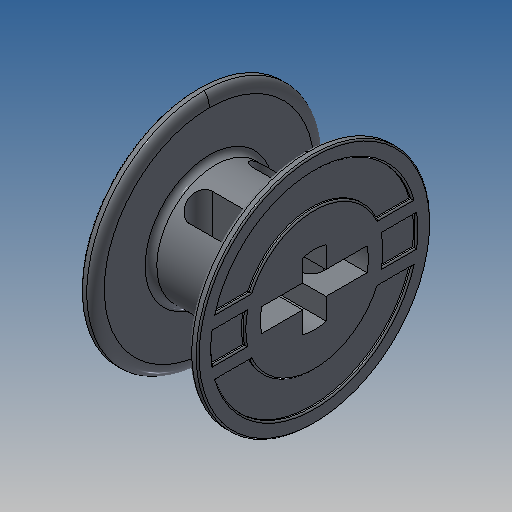
# Autodesk Inventor part: 61510-LtBluishGray
Saved by Autodesk Inventor 2025 (Build 290162010, 162A)
## iProperties
Created: 2014-10-31
Part Number: 61510-LtBluishGray
Material: ABS Plastic
Document SubType Name: Modeling
Designer: D. Kohfeld
Density: 1.06 g/cm^3
Appearance: LtBluishGray
Mass: 0.428094 g
Surface Area: 11.3807 cm^2
Volume: 0.403862 cm^3
Author: D. Kohfeld
Autodesk Inventor part; units mm, degrees
ref_plane "YZ Plane" through (0, 0, 0) normal (1, 0, 0) x (0, 1, 0)
ref_plane "XZ Plane" through (0, 0, 0) normal (0, 1, 0) x (-1, 0, 0)
ref_plane "XY Plane" through (0, 0, 0) normal (0, 0, 1) x (1, 0, 0)
sketch "Sketch2" plane through (0, 0, 0) normal (0, 0, 1) x (1, 0, 0)
  line L0 (-4, 8) -> (-4, 7)
  line L1 (-4, 7) -> (-3.8, 7)
  line L2 (-3.8, 7) -> (-3.8, 4.8)
  line L3 (-3.8, 4.8) -> (-4, 4.8)
  line L4 (-4, 4.8) -> (-4, 0)
  line L5 (-4, 0) -> (4, 0)
  line L6 (4, 0) -> (4, 4.8)
  line L7 (4, 4.8) -> (3.8, 4.8)
  line L8 (3.8, 4.8) -> (3.8, 7)
  line L9 (3.8, 7) -> (4, 7)
  line L10 (4, 7) -> (4, 8)
  line L11 (4, 8) -> (3.6, 8)
  line L12 (3.2, 7.2) -> (3.2, 4.4)
  arc A0 (2.8, 4) -> (3.2, 4.4) centre (2.8, 4.4) ccw
  line L13 (2.8, 4) -> (-2.8, 4)
  arc A1 (-3.2, 4.4) -> (-2.8, 4) centre (-2.8, 4.4) ccw
  line L14 (-3.2, 4.4) -> (-3.2, 7.2)
  line L15 (-3.6, 8) -> (-4, 8)
  ellipse E0 centre (-3.6, 7.2) end of major axis (-3.6, 8) minor radius 0.4 (-3.2, 7.2) -> (-3.6, 8) ccw
  ellipse E1 centre (3.6, 7.2) end of major axis (3.6, 8) minor radius 0.4 (3.6, 8) -> (3.2, 7.2) ccw
  point P0 (0, 0)
  point P1 (0, 0)
  dimension "d0" = 16
  dimension "d1" = 8
  dimension "d2" = 0.2
  dimension "d3" = 9.6
  dimension "d4" = 14
  dimension "d5" = 0.8
  dimension "d6" = 8
  dimension "d7" = 0.4
  dimension "d8" = 0.8
  dimension "d9" = 0.8
  dimension "d10" = 0.4
  constraints: 32 end point, 12 parallel, 4 equal length, 4 horizontal alignment, 4 point on circle, 4 tangent, 4 vertical alignment, 3 vertical, 2 centre point, 2 collinear, 1 coincident, 1 equal radius, 1 midpoint, 1 perpendicular, 8 other
  measures "d0" diameter of L15 L5
  measures "d1" distance between parallel lines of L10 L0
  measures "d2" distance between parallel lines of L0 L2
  measures "d3" diameter of L3.end L5
  measures "d4" diameter of L0.end L5
  measures "d5" distance between parallel lines of L14 L0
  measures "d6" diameter of L13 L5
  measures "d7" distance from line of L15.start L0
  measures "d8" distance from line of L14.end L15
  measures "d9" distance between parallel lines of L12 L10
  measures "d10" radius of A1
revolve "Revolution1" add sketch "Sketch2" angle 360 about axis through (-4, 0, 0) along (1, 0, 0)
sketch "Sketch3" plane through (4, 0, 0) normal (1, 0, 0) x (0, 0, -1)
  circle A0 centre (0, 0) radius 4.8 projected
  circle A1 centre (0, 0) radius 2.4 construction
  line L0 (-0.8, 2.2627) -> (-0.8, 0.8)
  line L1 (-0.8, 0.8) -> (-3.6125, 0.8)
  line L2 (0.8, 2.2627) -> (0.8, 0.8)
  line L3 (0.8, 0.8) -> (3.6125, 0.8)
  line L4 (-0.8, -2.2627) -> (-0.8, -0.8)
  line L5 (-0.8, -0.8) -> (-3.6125, -0.8)
  line L6 (0.8, -2.2627) -> (0.8, -0.8)
  line L7 (0.8, -0.8) -> (3.6125, -0.8)
  arc A2 (-3.6125, 0.8) -> (-3.6125, -0.8) centre (0, 0) ccw
  arc A3 (3.6125, -0.8) -> (3.6125, 0.8) centre (0, 0) ccw
  arc A4 (0.8, 2.2627) -> (-0.8, 2.2627) centre (0, 0) ccw
  arc A5 (-0.8, -2.2627) -> (0.8, -2.2627) centre (0, 0) ccw
  circle A6 centre (0, 0) radius 7 projected
  line L8 (-4.6947, 1) -> (-6.9282, 1)
  line L9 (-4.3635, 2) -> (-6.7082, 2)
  line L10 (-4.6947, -1) -> (-6.9282, -1)
  line L11 (-4.3635, -2) -> (-6.7082, -2)
  line L12 (4.6947, -1) -> (6.9282, -1)
  line L13 (4.3635, -2) -> (6.7082, -2)
  line L14 (4.6947, 1) -> (6.9282, 1)
  line L15 (4.3635, 2) -> (6.7082, 2)
  dimension "d12" = 4.8
  dimension "d13" = 1.6
  dimension "d14" = 1.6
  dimension "d15" = 7.4
  dimension "d16" = 2
  dimension "d17" = 1
  constraints: 32 end point, 12 point on circle, 10 equal length, 8 parallel, 7 perpendicular, 5 centre point, 3 coincident, 3 concentric, 2 horizontal alignment, 1 vertical, 18 other
  measures "d12" diameter of A1
  measures "d13" distance between parallel lines of L2 L0
  measures "d14" distance between parallel lines of L1 L5
  measures "d15" diameter of A2
  measures "d16" distance between parallel lines of L12 L14
  measures "d17" distance between parallel lines of L15 L14
extrude "Extrusion1" cut sketch "Sketch3" against normal through all contours A4 L2 L3 A3 L7 L6 A5 L4 L5 A2 L1 L0
extrude "Extrusion2" add sketch "Sketch3" against normal up to next contours A0 L15 A6 L14 | L12 A6 L13 A0 | A0 L8 A6 L9 | L11 A6 L10 A0
mirror "Mirror1" about plane through (0, 0, 0) normal (1, 0, 0) of "Extrusion2"
sketch "Sketch4" plane through (0, 0, 0) normal (0, 1, 0) x (-1, 0, 0)
  line L0 (-1.6, 2.2) -> (1.6, 2.2) construction
  line L1 (-1.6, 1.4) -> (1.6, 1.4)
  line L2 (1.6, 3) -> (-1.6, 3)
  arc A0 (-1.6, 3) -> (-1.6, 1.4) centre (-1.6, 2.2) ccw
  arc A1 (1.6, 1.4) -> (1.6, 3) centre (1.6, 2.2) ccw
  line L3 (-1.6, -2.2) -> (1.6, -2.2) construction
  line L4 (-1.6, -3) -> (1.6, -3)
  line L5 (1.6, -1.4) -> (-1.6, -1.4)
  arc A2 (-1.6, -1.4) -> (-1.6, -3) centre (-1.6, -2.2) ccw
  arc A3 (1.6, -3) -> (1.6, -1.4) centre (1.6, -2.2) ccw
  line L6 (1.6, -2.2) -> (1.6, 2.2) construction
  point P0 (0, 0)
  point P1 (0, 2.2)
  point P2 (0, -2.2)
  point P3 (1.6, 0)
  dimension "d22" = 1.6
  dimension "d23" = 4.8
  dimension "d24" = 2.8
  constraints: 18 end point, 8 point on circle, 8 tangent, 4 centre point, 4 parallel, 3 midpoint, 1 equal radius, 1 horizontal, 1 horizontal alignment, 1 perpendicular, 1 vertical alignment
  measures "d22" diameter of A1
  measures "d24" distance between parallel lines of L5 L1
extrude "Extrusion3" cut sketch "Sketch4" along normal through all both and the other way through all
fillet "Fillet1" radius 0.1 34 edges at (4, -8, 0) (-4, -8, 0) (4, 7, 0) (4, 0, 7) (4, -7, 0) (4, 0, -7) (4, 2, 5.5358) (4, 4.8, 0) (4, 2, -5.5358) (4, 1, -5.8114) (4, -1, -5.8114) (4, 0, -4.8) (4, 0, 4.8) (4, -1, 5.8114) (4, 1, 5.8114) (4, -2, 5.5358) (4, -4.8, 0) (4, -2, -5.5358) (-4, 7, 0) (-4, 2, -5.5358) (-4, 4.8, 0) (-4, 2, 5.5358) (-4, 1, 5.8114) (-4, 0, 4.8) (-4, -1, 5.8114) (-4, 0, 7) (-4, -4.8, 0) (-4, -2, 5.5358) (-4, -7, 0) (-4, -2, -5.5358) (-4, -1, -5.8114) (-4, 0, -7) (-4, 1, -5.8114) (-4, 0, -4.8)
equation "\"d0\" = 2 * lu"
equation "\"d1\" = lu"
equation "\"d6\" = lu"
equation "\"d9\" = d5"
equation "\"d13\" = axlet"
equation "\"d14\" = d13"
equation "\"d22\" = wall"
equation "\"d23\" = kd"
equation "\"lu\" = 8"
equation "\"axlet\" = 1.6"
equation "\"wall\" = 1.6"
equation "\"kd\" = 4.8"
body "Solid1"
